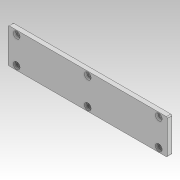
# Autodesk Inventor part: Link2_FlatCover
Saved by Autodesk Inventor 2020 (Build 240168000, 168)
## iProperties
Created: 2022-08-27
Part Number: Link2_FlatCover
Material: Generic
Document SubType Name: Modeling
Designer: DDeGo
Density: 1 g/cm^3
Appearance: Default
Author: DDeGo
Autodesk Inventor part; units mm, degrees
ref_plane "YZ Plane" through (0, 0, 0) normal (1, 0, 0) x (0, 1, 0)
ref_plane "XZ Plane" through (0, 0, 0) normal (0, 1, 0) x (-1, 0, 0)
ref_plane "XY Plane" through (0, 0, 0) normal (0, 0, 1) x (1, 0, 0)
sketch "Sketch1" plane through (0, 0, 0) normal (0, 0, 1) x (1, 0, 0)
  line L0 (-71, -15.75) -> (71, -15.75)
  line L1 (72, -14.75) -> (72, 14.75)
  line L2 (71, 15.75) -> (-71, 15.75)
  line L3 (-72, 14.75) -> (-72, -14.75)
  line L4 (-72, -15.75) -> (72, 15.75) construction
  line L5 (72, -15.75) -> (-72, 15.75) construction
  line L6 (0, 0) -> (0, 12) construction
  line L7 (0, 12) -> (64.25, 12) construction
  line L8 (0, 12) -> (-64.25, 12) construction
  line L9 (0, 0) -> (34.0768, 0) construction
  circle A0 centre (-64.25, 12) radius 1.75
  circle A1 centre (0, 12) radius 1.75
  circle A2 centre (64.25, 12) radius 1.75
  circle A3 centre (-64.25, -12) radius 1.75
  circle A4 centre (0, -12) radius 1.75
  circle A5 centre (64.25, -12) radius 1.75
  arc A6 (-71, 15.75) -> (-72, 14.75) centre (-71, 14.75) ccw
  arc A7 (72, 14.75) -> (71, 15.75) centre (71, 14.75) ccw
  arc A8 (71, -15.75) -> (72, -14.75) centre (71, -14.75) ccw
  arc A9 (-72, -14.75) -> (-71, -15.75) centre (-71, -14.75) ccw
  dimension "d0" = 144
  dimension "d1" = 31.5
  dimension "d2" = 64.25
  dimension "d3" = 12
  dimension "d4" = 3.5
  dimension "d5" = 1
  constraints: 20 end point, 10 centre point, 8 point on circle, 8 point on line, 8 tangent, 5 equal radius, 3 coincident, 3 horizontal, 3 symmetric about line, 2 midpoint, 2 parallel, 2 perpendicular, 1 collinear, 1 vertical, 3 other
  measures "d0" distance of L4.end L5.end
  measures "d1" distance of L5.start L4.end
  measures "d2" distance of L6.end L7.end
  measures "d3" distance between parallel lines of L9 L7
  measures "d4" diameter of A0
  measures "d5" radius of A6
extrude "Extrusion1" add sketch "Sketch1" along normal blind 4
sketch "Sketch2" plane through (0, 0, 4) normal (0, 0, 1) x (1, 0, 0)
  circle A0 centre (-64.25, 12) radius 1.75 projected
  circle A1 centre (-64.25, 12) radius 3
  circle A2 centre (0, 12) radius 1.75 projected
  circle A3 centre (0, 12) radius 3
  circle A4 centre (64.25, 12) radius 1.75 projected
  circle A5 centre (64.25, 12) radius 3
  circle A6 centre (64.25, -12) radius 1.75 projected
  circle A7 centre (64.25, -12) radius 3
  circle A8 centre (0, -12) radius 1.75 projected
  circle A9 centre (0, -12) radius 3
  circle A10 centre (-64.25, -12) radius 1.75 projected
  circle A11 centre (-64.25, -12) radius 3
  point P0 (0, 0)
  dimension "d8" = 6
  constraints: 6 centre point, 6 coincident, 5 equal radius
  measures "d8" diameter of A3
extrude "Extrusion2" cut sketch "Sketch2" against normal blind 2.2 contours A0 | A1 | A2 | A3 | A4 | A5 | A6 | A7 | A8 | A9 | A10 | A11
body "Solid1"
